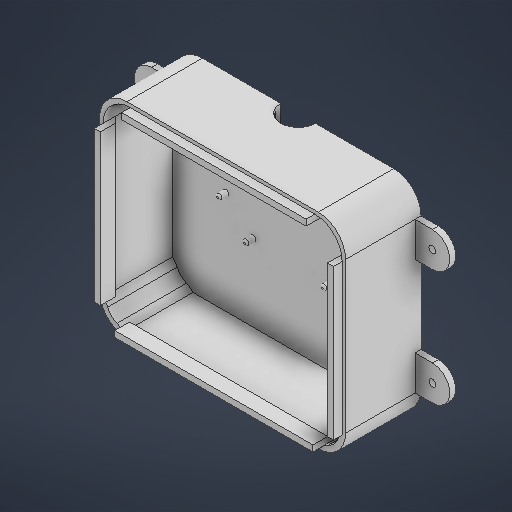
# Autodesk Inventor part: BreakerRear
Saved by Autodesk Inventor 2025.3 (Build 293356000, 356)
## iProperties
Created: 2026-02-28
Part Number: BreakerRear
Material: Generic
Document SubType Name: Modeling
Designer: Lemon
Density: 1 g/cm^3
Appearance: Default
Author: Lemon
Autodesk Inventor part; units mm, degrees
ref_plane "YZ Plane" through (0, 0, 0) normal (1, 0, 0) x (0, 1, 0)
ref_plane "XZ Plane" through (0, 0, 0) normal (0, 1, 0) x (-1, 0, 0)
ref_plane "XY Plane" through (0, 0, 0) normal (0, 0, 1) x (1, 0, 0)
sketch "Sketch1" plane through (0, 0, 0) normal (0, 0, 1) x (1, 0, 0)
  arc A0 (180, -20) -> (160, 0) centre (160, -20) ccw projected
  line L0 (20, 0) -> (160, 0) projected
  arc A1 (20, 0) -> (0, -20) centre (20, -20) ccw projected
  line L1 (0, -20) -> (0, -130) projected
  arc A2 (0, -130) -> (20, -150) centre (20, -130) ccw projected
  line L2 (20, -150) -> (160, -150) projected
  arc A3 (160, -150) -> (180, -130) centre (160, -130) ccw projected
  line L3 (180, -20) -> (180, -130) projected
  arc A4 (177.5, -132.5) -> (174.0625, -137.2496) centre (185.625, -141.9992) ccw projected
  arc A5 (167.2496, -144.0625) -> (174.0625, -137.2496) centre (162.5, -132.5) ccw projected
  arc A6 (167.2496, -144.0625) -> (162.5, -147.5) centre (171.9992, -155.625) ccw projected
  line L4 (162.5, -147.5) -> (17.5, -147.5) projected
  arc A7 (17.5, -147.5) -> (12.7504, -144.0625) centre (8.0008, -155.625) ccw projected
  arc A8 (5.9375, -137.2496) -> (12.7504, -144.0625) centre (17.5, -132.5) ccw projected
  arc A9 (5.9375, -137.2496) -> (2.5, -132.5) centre (-5.625, -141.9992) ccw projected
  line L5 (2.5, -132.5) -> (2.5, -22.5) projected
  arc A10 (22.5, -2.5) -> (2.5, -22.5) centre (22.5, -22.5) ccw projected
  line L6 (22.5, -2.5) -> (157.5, -2.5) projected
  arc A11 (177.5, -22.5) -> (157.5, -2.5) centre (157.5, -22.5) ccw projected
  line L7 (177.5, -22.5) -> (177.5, -132.5) projected
  point P0 (0, 0)
  point P1 (162.5, -147.5)
  point P2 (2.5, -132.5)
extrude "Extrusion1" add sketch "Sketch1" along normal blind 50.8
sketch "Sketch3" plane through (0, 0, 50.8) normal (0, 0, 1) x (1, 0, 0)
  line L0 (162.5, -147.5) -> (17.5, -147.5) projected
  line L1 (162.5, -147.5) -> (17.5, -147.5)
  line L2 (17.5, -147.5) -> (17.5, -143.055)
  line L3 (17.5, -143.055) -> (162.5, -143.055)
  line L4 (162.5, -143.055) -> (162.5, -147.5)
  line L5 (2.5, -132.5) -> (2.5, -22.5) projected
  line L6 (2.5, -132.5) -> (6.945, -132.5)
  line L7 (6.945, -132.5) -> (6.945, -22.5)
  line L8 (6.945, -22.5) -> (2.5, -22.5)
  line L9 (2.5, -22.5) -> (2.5, -132.5)
  arc A0 (22.5, -2.5) -> (2.5, -22.5) centre (22.5, -22.5) ccw projected
  line L10 (22.5, -2.5) -> (157.5, -2.5)
  line L11 (157.5, -2.5) -> (157.5, -6.945)
  line L12 (157.5, -6.945) -> (22.5, -6.945)
  line L13 (22.5, -6.945) -> (22.5, -2.5)
  line L14 (177.5, -22.5) -> (177.5, -132.5) projected
  line L15 (177.5, -132.5) -> (173.055, -132.5)
  line L16 (173.055, -132.5) -> (173.055, -22.5)
  line L17 (173.055, -22.5) -> (177.5, -22.5)
  line L18 (177.5, -22.5) -> (177.5, -132.5)
  point P0 (0, 0)
  point P1 (17.5, -147.5)
  dimension "d2" = 4.445
  dimension "d3" = 4.445
  dimension "d4" = 4.445
  dimension "d5" = 4.445
  constraints: 32 end point, 8 parallel, 4 horizontal, 4 perpendicular
  measures "d2" distance of L1.end L2.end
  measures "d3" distance of L8.end L7.end
  measures "d4" distance of L10.end L11.end
  measures "d5" distance of L16.end L17.end
extrude "Extrusion2" add sketch "Sketch3" along normal blind 6.35
sketch "Sketch4" plane through (0, 0, 50.8) normal (0, 0, -1) x (-1, 0, 0)
  line L0 (-6.945, -132.5) -> (-6.945, -22.5) projected
  line L1 (-2.5, -132.5) -> (-6.945, -132.5) projected
  line L2 (-2.5, -132.5) -> (-2.5, -22.5) projected
  line L3 (-6.945, -22.5) -> (-2.5, -22.5) projected
  line L4 (-22.5, -6.945) -> (-157.5, -6.945) projected
  line L5 (-22.5, -2.5) -> (-22.5, -6.945) projected
  line L6 (-22.5, -2.5) -> (-157.5, -2.5) projected
  line L7 (-157.5, -6.945) -> (-157.5, -2.5) projected
  line L8 (-162.5, -143.055) -> (-17.5, -143.055) projected
  line L9 (-162.5, -147.5) -> (-162.5, -143.055) projected
  line L10 (-162.5, -147.5) -> (-17.5, -147.5) projected
  line L11 (-17.5, -143.055) -> (-17.5, -147.5) projected
  line L12 (-173.055, -22.5) -> (-173.055, -132.5) projected
  line L13 (-177.5, -22.5) -> (-173.055, -22.5) projected
  line L14 (-177.5, -22.5) -> (-177.5, -132.5) projected
  line L15 (-173.055, -132.5) -> (-177.5, -132.5) projected
  point P0 (0, 0)
extrude "Extrusion3" add sketch "Sketch4" along normal blind 4.445
chamfer "Chamfer1" distance 4.445 angle 45 4 edges at (90, -147.5, 46.355) (2.5, -77.5, 46.355) (90, -2.5, 46.355) (177.5, -77.5, 46.355)
sketch "Sketch5" plane through (0, 0, 0) normal (0, 0, -1) x (-1, 0, 0)
  line L0 (0, -20) -> (0, -130) projected
  arc A0 (0, -20) -> (-20, 0) centre (-20, -20) ccw projected
  line L1 (-160, 0) -> (-20, 0) projected
  arc A1 (-160, 0) -> (-180, -20) centre (-160, -20) ccw projected
  line L2 (-180, -130) -> (-180, -20) projected
  arc A2 (-180, -130) -> (-160, -150) centre (-160, -130) ccw projected
  line L3 (-20, -150) -> (-160, -150) projected
  arc A3 (-20, -150) -> (0, -130) centre (-20, -130) ccw projected
  line L4 (-177.5, -22.5) -> (-177.5, -132.5) projected
  arc A4 (-157.5, -2.5) -> (-177.5, -22.5) centre (-157.5, -22.5) ccw projected
  line L5 (-22.5, -2.5) -> (-157.5, -2.5) projected
  arc A5 (-2.5, -22.5) -> (-22.5, -2.5) centre (-22.5, -22.5) ccw projected
  line L6 (-2.5, -132.5) -> (-2.5, -22.5) projected
  arc A6 (-2.5, -132.5) -> (-5.9375, -137.2496) centre (5.625, -141.9992) ccw projected
  arc A7 (-12.7504, -144.0625) -> (-5.9375, -137.2496) centre (-17.5, -132.5) ccw projected
  arc A8 (-12.7504, -144.0625) -> (-17.5, -147.5) centre (-8.0008, -155.625) ccw projected
  line L7 (-162.5, -147.5) -> (-17.5, -147.5) projected
  arc A9 (-162.5, -147.5) -> (-167.2496, -144.0625) centre (-171.9992, -155.625) ccw projected
  arc A10 (-174.0625, -137.2496) -> (-167.2496, -144.0625) centre (-162.5, -132.5) ccw projected
  arc A11 (-174.0625, -137.2496) -> (-177.5, -132.5) centre (-185.625, -141.9992) ccw projected
  line L8 (0, -130) -> (25.4, -130)
  line L9 (25.4, -130) -> (25.4, -104.6)
  line L10 (25.4, -104.6) -> (0, -104.6)
  line L11 (0, -104.6) -> (0, -130)
  line L12 (0, -20) -> (25.4, -20)
  line L13 (25.4, -20) -> (25.4, -45.4)
  line L14 (25.4, -45.4) -> (0, -45.4)
  line L15 (0, -45.4) -> (0, -20)
  line L16 (-180, -20) -> (-205.4, -20)
  line L17 (-205.4, -20) -> (-205.4, -45.4)
  line L18 (-205.4, -45.4) -> (-180, -45.4)
  line L19 (-180, -45.4) -> (-180, -20)
  line L20 (-180, -130) -> (-205.4, -130)
  line L21 (-205.4, -130) -> (-205.4, -104.6)
  line L22 (-205.4, -104.6) -> (-180, -104.6)
  line L23 (-180, -104.6) -> (-180, -130)
  dimension "d41" = 25.4
  dimension "d42" = 25.4
  dimension "d43" = 25.4
  dimension "d44" = 25.4
  dimension "d45" = 25.4
  dimension "d46" = 25.4
  dimension "d47" = 25.4
  dimension "d48" = 25.4
  constraints: 32 end point, 8 parallel, 4 horizontal, 4 perpendicular
  measures "d41" distance of L10.end L9.end
  measures "d42" distance of L9.end L8.end
  measures "d43" distance of L13.end L14.end
  measures "d44" distance of L12.end L13.end
  measures "d45" distance of L18.end L17.end
  measures "d46" distance of L17.end L16.end
  measures "d47" distance of L21.end L22.end
  measures "d48" distance of L20.end L21.end
extrude "Extrusion4" add sketch "Sketch5" along normal blind 4.445 contours L12 L13 L14 L0 | L0 A3 L3 A2 L2 A1 L1 A0 | L10 L9 L8 L0 | L2 L18 L17 L16 | L2 L20 L21 L22 | A4 L5 A5 L6 A6 A7 A8 L7 A9 A10 A11 L4
fillet "Fillet1" radius 12.7 8 edges at (205.4, -130, -2.2225) (205.4, -104.6, -2.2225) (205.4, -45.4, -2.2225) (205.4, -20, -2.2225) (-25.4, -45.4, -2.2225) (-25.4, -20, -2.2225) (-25.4, -104.6, -2.2225) (-25.4, -130, -2.2225)
sketch "Sketch7" plane through (0, 0, -4.445) normal (0, 0, -1) x (-1, 0, 0)
  arc A0 (-192.7, -104.6) -> (-192.7, -130) centre (-192.7, -117.3) ccw projected
  arc A1 (-192.7, -20) -> (-192.7, -45.4) centre (-192.7, -32.7) ccw projected
  arc A2 (12.7, -45.4) -> (12.7, -20) centre (12.7, -32.7) ccw projected
  arc A3 (12.7, -130) -> (12.7, -104.6) centre (12.7, -117.3) ccw projected
  constraints: 4 coincident
hole "Hole1" at (-12.7, -117.3, -4.445) at (-12.7, -32.7, -4.445) at (192.7, -32.7, -4.445) at (192.7, -117.3, -4.445) direction (0, 0, 1) diameter 5 end through all
sketch "Sketch10" plane through (20, 0, 50.8) normal (0, 1, 0) x (1, 0, 0)
  line L0 (140, 55.245) -> (0, 55.245) projected
  circle A0 centre (70, 55.245) radius 12.7
  point P0 (-20, 50.8)
  dimension "d49" = 25.4
  constraints: 1 centre point, 1 midpoint
  measures "d49" diameter of A0
extrude "Extrusion7" cut sketch "Sketch10" against normal blind 25.4
sketch "Sketch11" plane through (0, 0, 0) normal (0, 0, 1) x (1, 0, 0)
  circle A0 centre (138.26, -15.2) radius 2
  circle A1 centre (138.26, -72.1) radius 2
  line L0 (157.5, -2.5) -> (22.5, -2.5) projected
  line L1 (101.8967, -25.4) -> (78.1033, -25.4) projected
  line L2 (90, -25.4) -> (90, -30.603)
  circle A2 centre (41.74, -15.2) radius 2
  circle A3 centre (41.74, -72.1) radius 2
  circle A4 centre (61.55, -91.15) radius 2
  circle A5 centre (118.45, -91.15) radius 2
  point P0 (0, 0)
  dimension "d52" = 4
  dimension "d53" = 4
  dimension "d54" = 56.9
  dimension "d55" = 0
  dimension "d56" = 12.7
  dimension "d57" = 48.26
  dimension "d58" = 56.9
  dimension "d59" = 0
  dimension "d60" = 19.05
  dimension "d61" = 28.45
  constraints: 6 centre point, 2 end point, 2 midpoint, 2 symmetric about line, 1 vertical, 2 other
  measures "d52" diameter of A0
  measures "d53" diameter of A1
  measures "d54" distance of A1.centre A0.centre
  measures "d55" horizontal distance of A0.centre A1.centre
  measures "d56" distance from line of L0 A0.centre
  measures "d57" horizontal distance of L2.start A0.centre
  measures "d58" distance of A4.centre A5.centre
  measures "d59" vertical distance of A5.centre A4.centre
  measures "d60" vertical distance of A4.centre A3.centre
  measures "d61" horizontal distance of point (90, -25.4) A4.centre
extrude "Extrusion8" add sketch "Sketch11" along normal blind 6.35
fillet "Fillet2" radius 1.27 6 edges at (116.45, -91.15, 6.35) (136.26, -72.1, 6.35) (136.26, -15.2, 6.35) (59.55, -91.15, 6.35) (39.74, -72.1, 6.35) (39.74, -15.2, 6.35)
equation "\"d58\" = d54"
equation "\"d61\" = 0.5 * d58"
body "Solid1"
